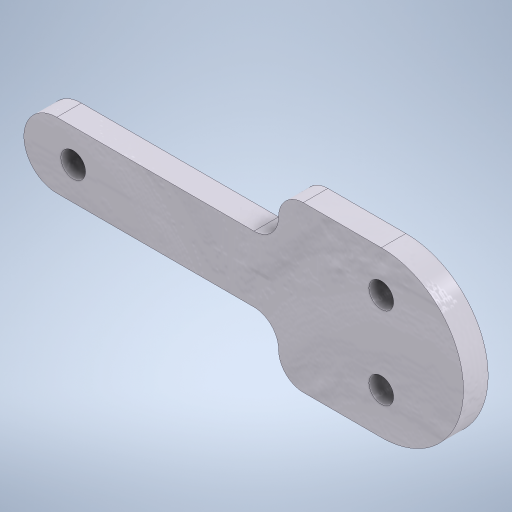
# Autodesk Inventor part: Arm5
Saved by Autodesk Inventor 2023 (Build 270158000, 158)
## iProperties
Created: 2024-02-06
Part Number: Arm5
Material: Aluminum 6061, Welded
Document SubType Name: Modeling
Designer: victo
Density: 2.7 g/cm^3
Appearance: Weld - Aluminum
Author: victo
Autodesk Inventor part; units mm, degrees
ref_plane "YZ Plane" through (0, 0, 0) normal (1, 0, 0) x (0, 1, 0)
ref_plane "XZ Plane" through (0, 0, 0) normal (0, 1, 0) x (-1, 0, 0)
ref_plane "XY Plane" through (0, 0, 0) normal (0, 0, 1) x (1, 0, 0)
sketch "Sketch1" plane through (0, 0, 0) normal (0, 0, 1) x (1, 0, 0)
  line L0 (0, 0) -> (37.5, 0) construction
  line L1 (0, -10) -> (37.5, -10)
  line L2 (37.5, 10) -> (0, 10)
  arc A0 (0, 10) -> (0, -10) centre (0, 0) ccw
  arc A1 (37.5, -10) -> (37.5, 10) centre (37.5, 0) ccw
  line L3 (0, 0) -> (37.5, 0) construction
  circle A2 centre (0, 0) radius 1.5
  circle A3 centre (37.5, -5) radius 1.5
  circle A4 centre (37.5, 5) radius 1.5
  point P0 (18.75, 0)
  dimension "d0" = 37.5
  dimension "d1" = 0
  dimension "d2" = 20
  dimension "d3" = 3
  dimension "d4" = 3
  dimension "d5" = 3
  dimension "d6" = 10
  dimension "d7" = 5
  dimension "d8" = 0
  dimension "d9" = 0
  constraints: 10 end point, 5 centre point, 4 point on circle, 4 tangent, 2 horizontal, 1 coincident, 1 collinear, 1 midpoint, 1 parallel
  measures "d0" distance of L0.start L0.end
  measures "d1" distance between parallel lines of L0 L3
  measures "d2" diameter of A1
  measures "d3" diameter of A2
  measures "d4" diameter of A3
  measures "d5" diameter of A4
  measures "d6" distance of A3.centre A4.centre
  measures "d7" distance from line of L1 A3.centre
  measures "d8" horizontal distance of L0.end A4.centre
  measures "d9" horizontal distance of L0.end A3.centre
extrude "Extrusion1" add sketch "Sketch1" along normal blind 3
sketch "Sketch2" plane through (0, 0, 0) normal (0, 0, -1) x (-1, 0, 0)
  line L0 (6, 4) -> (-25, 4)
  line L1 (-25, 10) -> (-25, -10)
  line L2 (-25, -4) -> (6, -4)
  line L3 (6, -4) -> (6, 4)
  arc A0 (-37.5, 10) -> (-37.5, -10) centre (-37.5, 0) ccw projected
  line L4 (0, -10) -> (-37.5, -10) projected
  arc A1 (0, -10) -> (0, 10) centre (0, 0) ccw projected
  line L5 (-37.5, 10) -> (0, 10) projected
  circle A2 centre (-37.5, 5) radius 1.5 projected
  circle A3 centre (-37.5, -5) radius 1.5 projected
  circle A4 centre (0, 0) radius 1.5 projected
  dimension "d12" = 6
  dimension "d13" = 4
  dimension "d14" = 4
  dimension "d15" = 25
  constraints: 8 end point, 4 point on line, 2 parallel, 1 horizontal, 1 perpendicular
  measures "d12" distance from line of point (0, 0) L3
  measures "d13" distance from line of L0 point (0, 0)
  measures "d14" distance from line of L2 point (0, 0)
  measures "d15" distance from line of point (0, 0) L1
extrude "Extrusion2" cut sketch "Sketch2" against normal up to surface (3 mm away) contours L0 L1 L5 A1 L4 L2 L3
fillet "Fillet1" radius 3 4 edges at (25, 4, 1.5) (25, 10, 1.5) (25, -4, 1.5) (25, -10, 1.5)
fillet "Fillet2" radius 4 2 edges at (-6, 4, 1.5) (-6, -4, 1.5)
body "Solid1"
